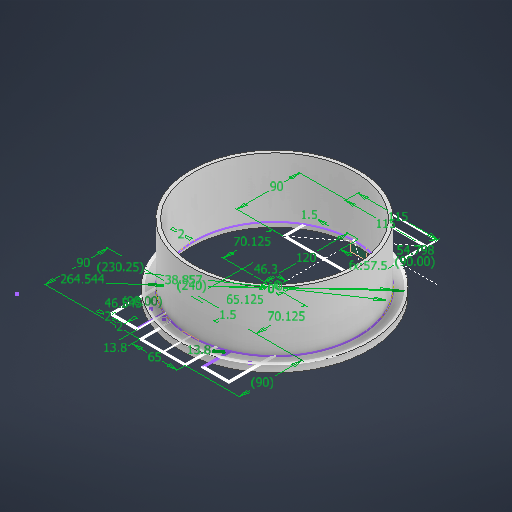
# Autodesk Inventor part: CoverHolder_Both
Saved by Autodesk Inventor 2026 (Build 300175000, 175)
## iProperties
Created: 2025-05-08
Part Number: CoverHolder_Both
Material: Generic
Document SubType Name: Modeling
Designer: Charl
Density: 1 g/cm^3
Appearance: Default
Author: Charl
Autodesk Inventor part; units mm, degrees
ref_plane "YZ Plane" through (0, 0, 0) normal (1, 0, 0) x (0, 1, 0)
ref_plane "XZ Plane" through (0, 0, 0) normal (0, 1, 0) x (-1, 0, 0)
ref_plane "XY Plane" through (0, 0, 0) normal (0, 0, 1) x (1, 0, 0)
sketch "l" plane through (0, 0, 0) normal (0, 1, 0) x (-1, 0, 0)
  circle A0 centre (0, 0) radius 120
  circle A1 centre (0, 0) radius 135
  point P0 (0, 120)
  point P1 (0, -120)
  point P2 (0, -135)
  point P3 (0, 135)
  dimension "d0" = 240
  dimension "d1" = 270
  constraints: 4 point on circle, 3 coincident, 2 centre point
  measures "d0" diameter of A0
  measures "d1" diameter of A1
extrude "Extrusion1" add sketch "l" along normal blind 10
sketch "Sketch2" plane through (0, 10, 0) normal (0, 1, 0) x (1, 0, 0)
  circle A0 centre (0, 0) radius 115.125
  circle A1 centre (0, 0) radius 120
  dimension "d4" = 230.25
  constraints: 2 centre point, 2 coincident
  measures "d4" diameter of A0
extrude "Extrusion2" add sketch "Sketch2" along normal blind 85.5
ref_plane "Work Plane1" through (0, 0, 120) normal (0, 0, 1) x (1, 0, 0)
ref_plane "Work Plane2" through (0, 0, -120) normal (0, 0, -1) x (-1, 0, 0)
sketch "Sketch3" plane through (0, 10, 0) normal (0, 1, 0) x (1, 0, 0)
  circle A0 centre (0, 0) radius 115.125 construction
  line L0 (0, 0) -> (0, 120) construction
  circle A1 centre (0, 0) radius 120 construction
  line L1 (0, 120) -> (57.5, 120) construction
  line L2 (57.5, 120) -> (57.5, 174.798)
  line L3 (57.5, 120) -> (112.298, 120) construction
  line L4 (57.5, 174.798) -> (-57.5, 174.798)
  line L5 (-57.5, 174.798) -> (-57.5, 120)
  dimension "d7" = 120
  dimension "d8" = 54.798
  dimension "d9" = 90
  dimension "d10" = 115
  dimension "d11" = 57.5
  constraints: 12 end point, 3 horizontal, 2 perpendicular, 2 vertical, 1 point on line, 1 vertical alignment
  measures "d7" distance of L0.start L0.end
  measures "d8" distance of L1.end L2.end
  measures "d9" angle of L3 L2
  measures "d10" distance of L2.end L4.end
  measures "d11" distance of L0.end L1.end
sketch "Sketch4" plane through (0, 10, 0) normal (0, 1, 0) x (1, 0, 0)
  line L0 (-32.5, -70.125) -> (32.5, -70.125)
  line L1 (32.5, -70.125) -> (32.5, -160.125)
  line L2 (32.5, -160.125) -> (-32.5, -160.125)
  line L3 (-32.5, -160.125) -> (-32.5, -70.125)
  circle A0 centre (0, 0) radius 115.125
  line L4 (31, -71.625) -> (-31, -71.625)
  line L5 (-31, -71.625) -> (-31, -158.625)
  line L6 (-31, -158.625) -> (31, -158.625)
  line L7 (31, -158.625) -> (31, -71.625)
  arc A1 (-32.5, -118.935) -> (-46.2997, -118.8397) centre (-39.3993, -118.814) ccw
  arc A2 (46.2999, -118.8962) -> (32.5, -118.8521) centre (39.3999, -118.8962) ccw
  circle A3 centre (0, 0) radius 120
  circle A4 centre (0, 0) radius 120
  line L8 (-85.1567, -65.125) -> (-46.2997, -65.125)
  line L9 (-46.2997, -65.125) -> (-46.2997, -126.0372)
  line L10 (-85.1567, -103.8141) -> (-85.1567, -65.125)
  circle A5 centre (0, 0) radius 134.2722
  line L11 (0, -71.625) -> (0, -158.625)
  line L12 (-83.1567, -108.9509) -> (-83.1567, -67.125)
  line L13 (-83.1567, -67.125) -> (-48.0393, -67.125)
  line L14 (-48.0393, -67.125) -> (-48.0393, -125.3844)
  circle A6 centre (0, 0) radius 132.2722
  circle A7 centre (0, 0) radius 115.125
  line L15 (-85.1567, -103.8141) -> (-85.1567, -150.3591)
  line L16 (-85.1567, -103.8141) -> (-38.6117, -103.8141) construction
  line L17 (-85.1567, -150.3591) -> (-46.2997, -150.3591)
  line L18 (-46.2997, -150.3591) -> (-46.2997, -126.0372)
  line L19 (-48.0393, -125.3844) -> (-48.0393, -148.3591)
  line L20 (-48.0393, -148.3591) -> (-83.1567, -148.3591)
  line L21 (-83.1567, -148.3591) -> (-83.1567, -108.9509)
  line L22 (46.2997, -65.125) -> (46.2999, -126.0371)
  line L23 (48.0393, -67.125) -> (48.0393, -125.3844)
  line L24 (85.1567, -65.125) -> (46.2997, -65.125)
  line L25 (83.1567, -67.125) -> (48.0393, -67.125)
  line L26 (83.1567, -108.9509) -> (83.1567, -67.125)
  line L27 (85.1567, -103.8141) -> (85.1567, -65.125)
  line L28 (85.1567, -103.8141) -> (85.1567, -150.3591)
  line L29 (83.1567, -148.3591) -> (83.1567, -108.9509)
  line L30 (85.1567, -150.3591) -> (46.2997, -150.3591)
  line L31 (48.0393, -148.3591) -> (83.1567, -148.3591)
  line L32 (46.2997, -150.3591) -> (46.2999, -126.0371)
  line L33 (48.0393, -125.3844) -> (48.0393, -148.3591)
  line L34 (57.5, 70.125) -> (-57.5, 70.125)
  line L35 (-57.5, 70.125) -> (-57.5, 160.125)
  line L36 (-57.5, 160.125) -> (57.5, 160.125)
  line L37 (57.5, 160.125) -> (57.5, 70.125)
  line L38 (57.5, 70.125) -> (-57.5, 160.125) construction
  line L39 (-57.5, 70.125) -> (57.5, 160.125) construction
  line L40 (-56, 158.625) -> (-56, 71.625)
  line L41 (-56, 71.625) -> (56, 71.625)
  line L42 (56, 71.625) -> (56, 158.625)
  line L43 (56, 158.625) -> (-56, 158.625)
  point P0 (0, 0)
  point P1 (-175.3676, -192.3287)
  point P2 (0, -115.125)
  point P3 (0, -70.125)
  point P4 (37.7289, -108.0229)
  point P5 (-27.2711, -108.0229)
  point P6 (36.2289, -108.4533)
  point P7 (-25.7711, -108.4533)
  point P8 (-61.2997, -115.125)
  point P9 (75.8883, -110.77)
  point P10 (37.7289, -113.0957)
  point P11 (37.7289, -118.7724)
  point P12 (-41.0708, -118.8403)
  point P13 (-27.2711, -118.7724)
  point P14 (-27.2711, -113.0957)
  point P15 (-42.8104, -107.5452)
  point P16 (-42.8104, -120.8208)
  point P17 (-77.9278, -100.4441)
  point P18 (-77.9278, -84.0963)
  point P19 (-79.9278, -82.1284)
  point P20 (-42.8104, -102.2037)
  point P21 (-77.9278, -77.1967)
  point P22 (-25.7711, -126.1688)
  point P23 (36.2289, -126.1688)
  point P24 (-27.2711, -127.8602)
  point P25 (37.7289, -127.8602)
  point P26 (-25.7711, -113.5073)
  point P27 (36.2289, -113.5073)
  point P28 (37.7289, -125.7979)
  point P29 (-27.2711, -125.7979)
  point P30 (53.2682, -107.5452)
  point P31 (51.5286, -118.8403)
  point P32 (90.3856, -82.1284)
  point P33 (88.3856, -84.0963)
  point P34 (90.3856, -101.3947)
  point P35 (53.2682, -122.965)
  point P36 (88.3856, -103.0035)
  point P37 (-77.9278, -103.0035)
  point P38 (53.2682, -102.2037)
  point P39 (0, 115.125)
  point P40 (0, 70.125)
  point P41 (-52.2711, 123.7569)
  point P42 (-50.7711, 124.4564)
  point P43 (61.2289, 124.4564)
  point P44 (62.7289, 123.7569)
  point P45 (61.2289, 103.0066)
  point P46 (62.7289, 102.1567)
  point P47 (-52.2711, 102.1567)
  point P48 (-50.7711, 103.0066)
  point P49 (61.2289, 108.5514)
  point P50 (-50.7711, 108.5514)
  dimension "d23" = 230.25
  dimension "d12" = 65
  dimension "d13" = 1.5
  dimension "d14" = 13.8
  dimension "d15" = 240
  dimension "d16" = 2
  dimension "d17" = 38.857
  dimension "d18" = 2
  dimension "d19" = 46.545
  dimension "d20" = 90
  dimension "d21" = 2
  dimension "d22" = 264.5444
  dimension "d24" = 13.7997
  dimension "d25" = 46.2997
  dimension "d26" = 90
  dimension "d27" = 65.125
  dimension "d28" = 70.125
  dimension "d29" = 90
  dimension "d30" = 115
  dimension "d31" = 1.5
  dimension "d32" = 70.125
  dimension "d33" = 90
  dimension "d34" = 0
  dimension "d35" = 0
  dimension "d36" = 0
  dimension "d37" = 0
  constraints: 88 end point, 12 perpendicular, 11 symmetric about line, 10 parallel, 9 point on circle, 7 centre point, 6 midpoint, 5 coincident, 4 horizontal, 4 vertical alignment, 2 point on line, 1 horizontal alignment, 1 tangent, 1 vertical, 10 other
  measures "d12" distance of L1.end L2.end
  measures "d13" distance between parallel lines of L0 L4
  measures "d14" diameter of A2
  measures "d15" diameter of A4
  measures "d16" radial gap between concentric circles of A5 A6
  measures "d17" distance of L8.start L8.end
  measures "d18" distance between parallel lines of L12 L10
  measures "d19" distance of L10.start L15.end
  measures "d20" angle of L15 L16
  measures "d21" distance between parallel lines of L17 L20
  measures "d22" diameter of A6
  measures "d24" distance between parallel lines of L3 L18
  measures "d25" distance from line of L9 A3.centre
  measures "d26" distance of L2.end L0.start
  measures "d27" distance from line of A4.centre L8
  measures "d28" distance from line of point (0, 0) L0
  measures "d29" distance of L0.end L1.end
  measures "d30" distance of L35.end L36.end
  measures "d31" distance between parallel lines of L35 L40
  measures "d32" vertical distance of L34.end point (0, 0)
  measures "d33" distance of L34.end L35.end
  measures "d34" distance of point (0, 0) A4.centre
  measures "d35" distance of point (0, 0) point (0, 0)
  measures "d36" distance of point (0, 0) A6.centre
  measures "d37" distance of point (0, 0) A3.centre
equation "\"d11\" = 0.5 * d10"
body "Solid1"
